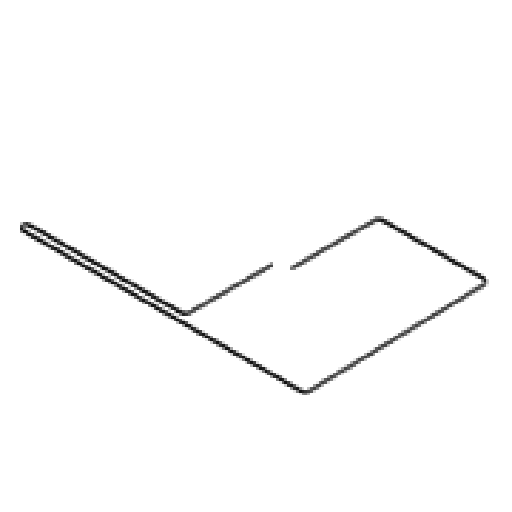
# Autodesk Inventor part: Belt_1
Saved by Autodesk Inventor 2023.2 (Build 272271000, 271)
## iProperties
Created: 2023-02-04
Part Number: Belt_1
Material: Rubber
Document SubType Name: Modeling
Designer: remop
Density: 0.93 g/cm^3
Appearance: Rubber - Black
Author: remop
Autodesk Inventor part; units mm, degrees
ref_plane "YZ Plane" through (0, 0, 0) normal (1, 0, 0) x (0, 1, 0)
ref_plane "XZ Plane" through (0, 0, 0) normal (0, 1, 0) x (-1, 0, 0)
ref_plane "XY Plane" through (0, 0, 0) normal (0, 0, 1) x (1, 0, 0)
sketch "Sketch1" plane through (0, 0, 0) normal (0, 1, 0) x (-1, 0, 0)
  circle A0 centre (146.7383, -31.3394) radius 6.1 projected
  circle A1 centre (146.7383, -31.3394) radius 7.5 projected
  circle A2 centre (-107.7617, -44.8394) radius 7.5 projected
  circle A3 centre (-107.7617, -44.8394) radius 6 projected
  circle A4 centre (-142.7617, -335.2394) radius 7.5 projected
  circle A5 centre (-142.7617, -335.2394) radius 6 projected
  circle A6 centre (-314.7617, -335.1394) radius 7.5 projected
  circle A7 centre (-314.7617, -335.1394) radius 6.1 projected
  circle A8 centre (-322.7617, -31.3394) radius 7.5 projected
  circle A9 centre (-322.7617, -31.3394) radius 6.1 projected
  line L0 (-322.7617, -23.8394) -> (146.7383, -23.8394)
  line L1 (146.7383, -38.8394) -> (-107.7617, -38.8394)
  line L2 (-107.7587, -37.3394) -> (146.7359, -37.4394)
  line L3 (146.7383, -25.2394) -> (-322.7617, -25.2394)
  line L4 (-328.8595, -31.5) -> (-320.8595, -335.3)
  line L5 (-322.2591, -335.3369) -> (-330.2591, -31.5369)
  line L6 (-314.7617, -341.2394) -> (-142.7617, -341.2394)
  line L7 (-142.766, -342.7394) -> (-314.766, -342.6394)
  line L8 (-115.2617, -44.8394) -> (-115.2617, -185.0394)
  line L9 (-115.2617, -185.0394) -> (-113.7617, -185.0394)
  line L10 (-113.7617, -185.0394) -> (-113.7617, -44.8394)
  line L11 (-136.7617, -335.2394) -> (-136.7617, -195.0394)
  line L12 (-136.7617, -195.0394) -> (-135.2617, -195.0394)
  line L13 (-135.2617, -195.0394) -> (-135.2617, -335.2394)
  arc A10 (-100.7617, -192.5394) -> (-100.7617, -187.5394) centre (-96.4315, -190.0394) ccw
  point P0 (0, 0)
  point P1 (-147.2617, -341.2394)
  constraints: 28 end point, 22 point on circle, 22 tangent, 3 perpendicular, 2 vertical, 1 centre point, 1 parallel, 4 other
extrude "Extrusion1" add sketch "Sketch1" against normal blind 6 contours A0 L3 A1 L2 | L3 A8 L0 A1 | A1 L1 A2 L2 | L3 A9 L4 A8 | A2 L1 A3 L10 | A2 L10 L9 L8 | A8 L4 A6 L5 | A6 L4 A7 L6 | A6 L6 A4 L7 | A4 L6 A5 L11 | A4 L11 L12 L13 picked at (144.276, -37.6941) picked at (-329.0502, -33.966) picked at (-114.0352, -47.3793) picked at (-312.3021, -341.4951) picked at (-136.4882, -332.6995)
body "Solid1"
